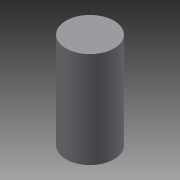
# Autodesk Inventor part: Pin_B_1.5mm_Piston
Saved by Autodesk Inventor 2015 (Build 190159000, 159)
## iProperties
Created: 2016-07-06
Part Number: Pin_B_1.5mm_Piston
Material: Generic
Document SubType Name: Modeling
Designer: Neelotpal Nag
Density: 1 g/cm^3
Appearance: Default
Author: Neelotpal Nag
Autodesk Inventor part; units mm, degrees
ref_plane "YZ Plane" through (0, 0, 0) normal (1, 0, 0) x (0, 1, 0)
ref_plane "XZ Plane" through (0, 0, 0) normal (0, 1, 0) x (-1, 0, 0)
ref_plane "XY Plane" through (0, 0, 0) normal (0, 0, 1) x (1, 0, 0)
sketch "Sketch1" plane through (0, 0, 0) normal (0, 0, 1) x (1, 0, 0)
  circle A0 centre (0, 0) radius 0.75
  dimension "d0" = 1.5
  constraints: 1 centre point, 1 coincident
  measures "d0" diameter of A0
extrude "Extrusion1" add sketch "Sketch1" along normal mid plane 3
body "Solid1"
